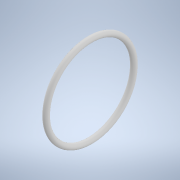
# Autodesk Inventor part: RD013
Saved by Autodesk Inventor 2021 (Build 250183000, 183)
## iProperties
Created: 2020-11-01
Part Number: RD013
Material: 一般
Document SubType Name: Modeling
Designer: ryusei
Density: 1 g/cm^3
Appearance: 既定
Author: ryusei
Title: オーリング
Autodesk Inventor part; units mm, degrees
ref_plane "YZ Plane" through (0, 0, 0) normal (1, 0, 0) x (0, 1, 0)
ref_plane "XZ Plane" through (0, 0, 0) normal (0, 1, 0) x (-1, 0, 0)
ref_plane "XY Plane" through (0, 0, 0) normal (0, 0, 1) x (1, 0, 0)
sketch "スケッチ4" plane through (0, 0, 0) normal (0, 0, 1) x (1, 0, 0)
  circle A0 centre (0, 24) radius 1.5
  line L0 (0, 0) -> (2.5034, 0)
  dimension "d15" = 3
  dimension "d16" = 24
  constraints: 2 end point, 1 centre point, 1 horizontal
  measures "d15" diameter of A0
  measures "d16" distance of L0.start A0.centre
revolve "回転2" add sketch "スケッチ4" angle 360 about axis through (0, 0, 0) along (1, 0, 0)
